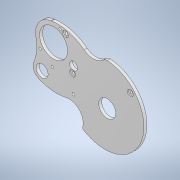
# Autodesk Inventor part: 足内フレーム
Saved by Autodesk Inventor 2022.2 (Build 262287030, 287C)
## iProperties
Created: 2022-01-10
Part Number: 足内フレーム
Material: Aluminum 2014-T4
Document SubType Name: Modeling
Designer: acps
Density: 2.8 g/cm^3
Appearance: Satin
Author: acps
Autodesk Inventor part; units mm, degrees
ref_plane "YZ Plane" through (0, 0, 0) normal (1, 0, 0) x (0, 1, 0)
ref_plane "XZ Plane" through (0, 0, 0) normal (0, 1, 0) x (-1, 0, 0)
ref_plane "XY Plane" through (0, 0, 0) normal (0, 0, 1) x (1, 0, 0)
sketch "Sketch2" plane through (0, 0, 0) normal (0, 0, 1) x (1, 0, 0)
  circle A0 centre (46.4683, 30) radius 14
  circle A1 centre (66.4734, 20) radius 20.5 construction
  circle A2 centre (100, 0) radius 30 construction
  circle A3 centre (123.045, 25) radius 1.25
  circle A4 centre (100, 0) radius 3 construction
  circle A5 centre (35, 0) radius 6.025
  circle A6 centre (35, 0) radius 9
  arc A7 (26.7096, 3.5028) -> (28.866, 26.2368) centre (-8.2942, 18.2924) ccw
  arc A8 (44, 47.83) -> (28.866, 26.2368) centre (46.4683, 30) ccw
  arc A9 (110.6259, 39.2116) -> (45.1112, 47.9488) centre (57.174, -111.5959) ccw construction
  arc A10 (91.0837, -36) -> (110.6259, 39.2116) centre (97.597, 2.4523) ccw
  arc A11 (28.683, 27.2278) -> (91.0837, -36) centre (103.7763, 38.9326) ccw construction
  circle A12 centre (58.3063, 43.4) radius 1.5
  arc A13 (44.5539, 47.9057) -> (44, 47.83) centre (65.9403, -110.6586) ccw
  arc A14 (76.7854, 39.1678) -> (44.5539, 47.9057) centre (50.3015, 5.2915) ccw
  arc A15 (76.7854, 39.1678) -> (96.2775, 40.0369) centre (86.0239, 50.9851) ccw
  arc A16 (100.004, 41.3779) -> (96.2775, 40.0369) centre (99.6954, 36.3875) ccw
  arc A17 (91.0837, -36) -> (100.004, 41.3779) centre (97.597, 2.4523) ccw
  arc A18 (75.52, -28.3291) -> (58.8706, -11.0424) centre (62.0019, -24.6877) ccw
  arc A19 (31.2271, -8.171) -> (58.8706, -11.0424) centre (49.2531, 30.8683) ccw
  arc A20 (75.52, -28.3291) -> (76.4189, -30.5623) centre (77.4512, -28.8493) ccw
  arc A21 (76.4189, -30.5623) -> (91.0837, -36) centre (98.098, 5.4101) ccw
  circle A22 centre (58.3063, 43.4) radius 1.5
  circle A23 centre (123.045, 25) radius 1.25
  circle A24 centre (100, 0) radius 3 construction
  circle A25 centre (100, 0) radius 8.525
  circle A26 centre (65.359, 13) radius 1.25
  arc A27 (131.5793, 3.5511) -> (107.9544, 34.8363) centre (97.597, 2.4523) ccw construction
  circle A28 centre (66.4734, 20) radius 4
  circle A29 centre (66.299, -4.4994) radius 4 construction
  circle A30 centre (66.299, -4.4994) radius 1.5
  circle A31 centre (66.299, -4.4994) radius 3 construction
  circle A32 centre (53.0056, 45.2) radius 1.25
  arc A33 (59.6568, 44.1821) -> (46.2779, 45.0886) centre (50.3015, 5.2915) ccw construction
  circle A34 centre (45.1, 8.5) radius 1.25
  circle A35 centre (33, 18) radius 1.25
  arc A36 (31.0568, 25.3067) -> (30.8433, 25.9979) centre (-68.6067, -5.1096) ccw construction
  line L0 (51.7556, 0) -> (32.0278, 0) construction
  point P0 (0, 0)
  point P1 (0, 0)
  point P2 (86.6921, 36)
  point P3 (61.5525, 46.7935)
  point P4 (110.6259, 39.2116)
  dimension "d0" = 12.05
  dimension "d1" = 18
  dimension "d4" = 4
  dimension "d6" = 15
  dimension "d7" = 14
  dimension "d8" = 2
  dimension "d9" = 43
  dimension "d10" = 5
  dimension "d11" = 43
  dimension "d12" = 36
  dimension "d13" = 44
  dimension "d14" = 42
  dimension "d15" = 74
  dimension "d16" = 118
  dimension "d18" = 110.6259
  dimension "d21" = 17.05
  dimension "d22" = 2.5
  dimension "d23" = 37
  dimension "d24" = 13
  dimension "d26" = 3
  dimension "d27" = 2.5
  dimension "d28" = 25
  dimension "d29" = 5
  dimension "d35" = 8
  dimension "d36" = 8
  dimension "d37" = 3
  dimension "d38" = 6
  dimension "d39" = 2.5
  dimension "d40" = 3
  dimension "d42" = 45.2
  dimension "d43" = 2.5
  dimension "d44" = 8.5
  dimension "d45" = 45.1
  dimension "d46" = 2.5
  dimension "d50" = 65.359
  dimension "d51" = 35
  dimension "d52" = 38
  dimension "d53" = 18
  dimension "d54" = 33
  constraints: 41 point on circle, 36 centre point, 16 tangent, 8 coincident, 6 concentric, 2 end point, 2 horizontal, 1 point on line, 14 other
  measures "d0" diameter of A5
  measures "d1" diameter of A6
  measures "d4" radial gap between concentric circles of A8 A0
  measures "d6" radius of A15
  measures "d7" radius of A18
  measures "d8" radius of A20
  measures "d9" radius of A19
  measures "d10" radius of A16
  measures "d11" radius of A14
  measures "d12" vertical distance of point (0, 0) point (86.692, 36)
  measures "d13" horizontal distance of point (0, 0) A8.start
  measures "d14" radius of A21
  measures "d18" horizontal distance of point (0, 0) A10.end
  measures "d21" diameter of A25
  measures "d22" diameter of A26
  measures "d23" distance of A2.centre A26.centre
  measures "d24" vertical distance of point (0, 0) A26.centre
  measures "d26" diameter of A12
  measures "d27" diameter of A3
  measures "d28" vertical distance of point (0, 0) A3.centre
  measures "d29" radial gap between concentric circles of A10 A27
  measures "d35" diameter of A28
  measures "d36" diameter of A29
  measures "d37" diameter of A30
  measures "d38" diameter of A31
  measures "d39" diameter of A32
  measures "d40" radial gap between concentric circles of A14 A33
  measures "d42" vertical distance of point (0, 0) A32.centre
  measures "d43" diameter of A34
  measures "d44" vertical distance of point (0, 0) A34.centre
  measures "d45" horizontal distance of point (0, 0) A34.centre
  measures "d46" diameter of A35
  measures "d50" horizontal distance of point (0, 0) A26.centre
  measures "d51" distance of A6.centre point (0, 0)
  measures "d52" radius of A7
  measures "d53" vertical distance of point (0, 0) A35.centre
  measures "d54" horizontal distance of point (0, 0) A35.centre
extrude "Extrusion1" add sketch "Sketch2" against normal blind 3
sketch "Sketch3" plane through (0, 0, 0) normal (0, 0, 1) x (1, 0, 0)
  circle A0 centre (58.3063, 43.4) radius 3
  circle A1 centre (65.359, 13) radius 3
  circle A2 centre (123.045, 25) radius 1.25 projected
  circle A3 centre (123.045, 25) radius 3
  point P0 (0, 0)
  dimension "d30" = 6
  dimension "d31" = 6
  dimension "d32" = 6
  constraints: 3 centre point, 3 coincident
  measures "d30" diameter of A0
  measures "d31" diameter of A1
  measures "d32" diameter of A3
extrude "Extrusion2" cut sketch "Sketch3" against normal blind 1 contours A0 | A1 | A2 | A3
body "Solid1"
